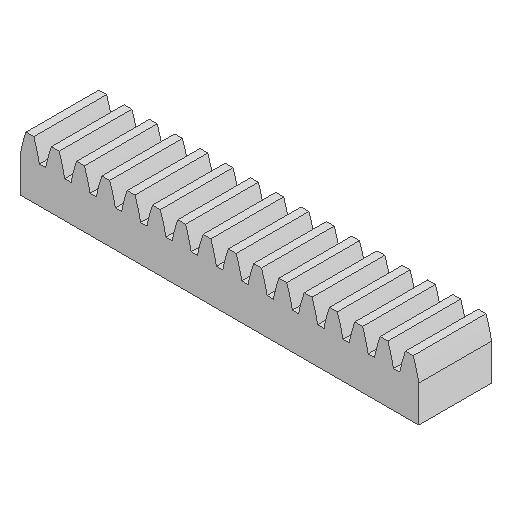
# Autodesk Inventor part: 1p10 DP3 gear attachment
Saved by Autodesk Inventor 2023 (Build 270158000, 158)
## iProperties
Created: 2023-03-02
Part Number: 1p10 DP3 gear attachment
Material: Generic
Document SubType Name: Modeling
Designer: Ethan Ko
Density: 1 g/cm^3
Appearance: Default
Author: Ethan Ko
Autodesk Inventor part; units mm, degrees
ref_plane "YZ Plane" through (0, 0, 0) normal (1, 0, 0) x (0, 1, 0)
ref_plane "XZ Plane" through (0, 0, 0) normal (0, 1, 0) x (-1, 0, 0)
ref_plane "XY Plane" through (0, 0, 0) normal (0, 0, 1) x (1, 0, 0)
sketch "Sketch1" plane through (0, 0, 0) normal (0, 0, 1) x (1, 0, 0)
  line L0 (0, 0) -> (1.071, 0)
  line L1 (0.5355, 0) -> (0.5355, -2.881)
  line L2 (0.5355, -2.881) -> (1.8385, -2.881)
  line L3 (1.8385, -2.881) -> (0.5355, -2.881)
  line L4 (0.5355, -2.881) -> (-0.7675, -2.881)
  arc A0 (0, 0) -> (-0.7675, -2.881) centre (20.5625, -7.0206) ccw
  arc A1 (1.8385, -2.881) -> (1.071, 0) centre (-19.4915, -7.0206) ccw
  line L5 (1.8385, -2.881) -> (2.7085, -2.881)
  line L6 (2.7085, -2.881) -> (5.3145, -2.881)
  line L7 (4.0115, -2.881) -> (4.0115, 0)
  line L8 (4.0115, 0) -> (3.476, 0)
  line L9 (4.0115, 0) -> (4.547, 0)
  arc A2 (3.476, 0) -> (2.7085, -2.881) centre (24.0385, -7.0206) ccw
  arc A3 (5.3145, -2.881) -> (4.547, 0) centre (-16.0155, -7.0206) ccw
  line L10 (5.3145, -2.881) -> (6.1845, -2.881)
  line L11 (6.1845, -2.881) -> (8.7905, -2.881)
  line L12 (7.4875, -2.881) -> (7.4875, 0)
  line L13 (7.4875, 0) -> (6.9515, 0)
  line L14 (7.4875, 0) -> (8.0235, 0)
  arc A4 (6.9515, 0) -> (6.1845, -2.881) centre (27.5152, -7.0172) ccw
  arc A5 (8.7905, -2.881) -> (8.0235, 0) centre (-12.5402, -7.0172) ccw
  line L15 (8.7905, -2.881) -> (9.6605, -2.881)
  line L16 (9.6605, -2.881) -> (12.2665, -2.881)
  line L17 (10.9635, -2.881) -> (10.9635, 0)
  line L18 (10.9635, 0) -> (10.4275, 0)
  line L19 (10.9635, 0) -> (11.4995, 0)
  arc A6 (10.4275, 0) -> (9.6605, -2.881) centre (30.9912, -7.0172) ccw
  arc A7 (12.2665, -2.881) -> (11.4995, 0) centre (-9.0642, -7.0172) ccw
  line L20 (-0.7675, -2.881) -> (-0.7675, -7.881)
  line L21 (12.2665, -2.881) -> (13.1365, -2.881)
  line L22 (13.1365, -2.881) -> (15.7425, -2.881)
  line L23 (14.4395, -2.881) -> (14.4395, 0)
  line L24 (14.4395, 0) -> (13.9035, 0)
  line L25 (14.4395, 0) -> (14.9755, 0)
  arc A8 (13.9035, 0) -> (13.1365, -2.881) centre (34.4672, -7.0172) ccw
  arc A9 (15.7425, -2.881) -> (14.9755, 0) centre (-5.5882, -7.0172) ccw
  line L26 (15.7425, -2.881) -> (16.6125, -2.881)
  line L27 (16.6125, -2.881) -> (19.2185, -2.881)
  line L28 (17.9155, -2.881) -> (17.9155, 0)
  line L29 (17.9155, 0) -> (17.3795, 0)
  line L30 (17.9155, 0) -> (18.4515, 0)
  arc A10 (17.3795, 0) -> (16.6125, -2.881) centre (37.9432, -7.0172) ccw
  arc A11 (19.2185, -2.881) -> (18.4515, 0) centre (-2.1122, -7.0172) ccw
  line L31 (19.2185, -2.881) -> (20.0885, -2.881)
  line L32 (20.0885, -2.881) -> (22.6945, -2.881)
  line L33 (21.3915, -2.881) -> (21.3915, 0)
  line L34 (21.3915, 0) -> (20.8555, 0)
  line L35 (21.3915, 0) -> (21.9275, 0)
  arc A12 (20.8555, 0) -> (20.0885, -2.881) centre (41.4192, -7.0172) ccw
  arc A13 (22.6945, -2.881) -> (21.9275, 0) centre (1.3638, -7.0172) ccw
  line L36 (22.6945, -2.881) -> (23.5645, -2.881)
  line L37 (23.5645, -2.881) -> (26.1705, -2.881)
  line L38 (24.8675, -2.881) -> (24.8675, 0)
  line L39 (24.8675, 0) -> (24.3315, 0)
  line L40 (24.8675, 0) -> (25.4035, 0)
  arc A14 (24.3315, 0) -> (23.5645, -2.881) centre (44.8952, -7.0172) ccw
  arc A15 (26.1705, -2.881) -> (25.4035, 0) centre (4.8398, -7.0172) ccw
  line L41 (26.1705, -2.881) -> (27.0405, -2.881)
  line L42 (27.0405, -2.881) -> (29.6465, -2.881)
  line L43 (29.6465, -2.881) -> (30.5165, -2.881)
  line L44 (30.5165, -2.881) -> (33.1225, -2.881)
  line L45 (33.1225, -2.881) -> (33.9925, -2.881)
  line L46 (33.9925, -2.881) -> (36.5985, -2.881)
  line L47 (36.5985, -2.881) -> (37.4685, -2.881)
  line L48 (37.4685, -2.881) -> (40.0745, -2.881)
  line L49 (40.0745, -2.881) -> (40.9445, -2.881)
  line L50 (40.9445, -2.881) -> (43.5505, -2.881)
  line L51 (43.5505, -2.881) -> (44.4205, -2.881)
  line L52 (44.4205, -2.881) -> (47.0265, -2.881)
  line L53 (47.0265, -2.881) -> (47.8965, -2.881)
  line L54 (47.8965, -2.881) -> (50.5025, -2.881)
  line L55 (50.5025, -2.881) -> (51.3725, -2.881)
  line L56 (51.3725, -2.881) -> (53.9785, -2.881)
  line L57 (53.9785, -2.881) -> (53.9785, -7.881)
  line L58 (53.9785, -7.881) -> (-0.7675, -7.881)
  line L59 (28.3435, -2.881) -> (28.3435, 0)
  line L60 (31.8195, -2.881) -> (31.8195, 0)
  line L61 (31.8195, 0) -> (31.2835, 0)
  line L62 (35.2955, -2.881) -> (35.2955, 0)
  line L63 (35.2955, 0) -> (34.7595, 0)
  line L64 (38.7715, -2.881) -> (38.7715, 0)
  line L65 (38.7715, 0) -> (38.2355, 0)
  line L66 (42.2475, -2.881) -> (42.2475, 0)
  line L67 (42.2475, 0) -> (41.7115, 0)
  line L68 (45.7235, -2.881) -> (45.7235, 0)
  line L69 (45.7235, 0) -> (45.1875, 0)
  line L70 (49.1995, -2.881) -> (49.1995, 0)
  line L71 (49.1995, 0) -> (48.6635, 0)
  line L72 (52.6755, -2.881) -> (52.6755, 0)
  line L73 (52.6755, 0) -> (52.1395, 0)
  line L74 (52.6755, 0) -> (53.2115, 0)
  line L75 (49.1995, 0) -> (49.7355, 0)
  line L76 (45.7235, 0) -> (46.2595, 0)
  line L77 (42.2475, 0) -> (42.7835, 0)
  line L78 (38.7715, 0) -> (39.3075, 0)
  line L79 (35.2955, 0) -> (35.8315, 0)
  line L80 (31.8195, 0) -> (32.3555, 0)
  line L81 (28.3435, 0) -> (28.8795, 0)
  line L82 (28.3435, 0) -> (27.8075, 0)
  arc A16 (27.8075, 0) -> (27.0405, -2.881) centre (48.3712, -7.0172) ccw
  arc A17 (29.6465, -2.881) -> (28.8795, 0) centre (8.3158, -7.0172) ccw
  arc A18 (31.2835, 0) -> (30.5165, -2.881) centre (51.8472, -7.0172) ccw
  arc A19 (33.1225, -2.881) -> (32.3555, 0) centre (11.7918, -7.0172) ccw
  arc A20 (34.7595, 0) -> (33.9925, -2.881) centre (55.3232, -7.0172) ccw
  arc A21 (36.5985, -2.881) -> (35.8315, 0) centre (15.2678, -7.0172) ccw
  arc A22 (38.2355, 0) -> (37.4685, -2.881) centre (58.7992, -7.0172) ccw
  arc A23 (40.0745, -2.881) -> (39.3075, 0) centre (18.7438, -7.0172) ccw
  arc A24 (41.7115, 0) -> (40.9445, -2.881) centre (62.2752, -7.0172) ccw
  arc A25 (43.5505, -2.881) -> (42.7835, 0) centre (22.2198, -7.0172) ccw
  arc A26 (45.1875, 0) -> (44.4205, -2.881) centre (65.7512, -7.0172) ccw
  arc A27 (47.0265, -2.881) -> (46.2595, 0) centre (25.6958, -7.0172) ccw
  arc A28 (48.6635, 0) -> (47.8965, -2.881) centre (69.2272, -7.0172) ccw
  arc A29 (50.5025, -2.881) -> (49.7355, 0) centre (29.1718, -7.0172) ccw
  arc A30 (52.1395, 0) -> (51.3725, -2.881) centre (72.7032, -7.0172) ccw
  arc A31 (53.9785, -2.881) -> (53.2115, 0) centre (32.6478, -7.0172) ccw
  dimension "d0" = 1.071
  dimension "d1" = 2.881
  dimension "d3" = 1.303
  dimension "d4" = 1.303
  dimension "d5" = 21.728
  dimension "d6" = 21.728
  dimension "d7" = 0.87
  dimension "d8" = 2.606
  dimension "d9" = 0.5355
  dimension "d10" = 0.5355
  dimension "d11" = 21.728
  dimension "d12" = 21.728
  dimension "d13" = 0.87
  dimension "d14" = 2.606
  dimension "d15" = 0.536
  dimension "d16" = 0.536
  dimension "d17" = 21.728
  dimension "d18" = 21.728
  dimension "d19" = 0.87
  dimension "d20" = 2.606
  dimension "d21" = 0.536
  dimension "d22" = 0.536
  dimension "d23" = 21.728
  dimension "d24" = 21.728
  dimension "d25" = 5
  dimension "d27" = 0.87
  dimension "d28" = 2.606
  dimension "d29" = 0.536
  dimension "d30" = 0.536
  dimension "d31" = 21.728
  dimension "d32" = 21.728
  dimension "d33" = 0.87
  dimension "d34" = 2.606
  dimension "d35" = 0.536
  dimension "d36" = 0.536
  dimension "d37" = 21.728
  dimension "d38" = 21.728
  dimension "d39" = 0.87
  dimension "d40" = 2.606
  dimension "d41" = 0.536
  dimension "d42" = 0.536
  dimension "d43" = 21.728
  dimension "d44" = 21.728
  dimension "d45" = 0.87
  dimension "d46" = 2.606
  dimension "d47" = 0.536
  dimension "d48" = 0.536
  dimension "d49" = 21.728
  dimension "d50" = 21.728
  dimension "d51" = 0.87
  dimension "d52" = 2.606
  dimension "d53" = 0.87
  dimension "d54" = 2.606
  dimension "d55" = 0.87
  dimension "d56" = 2.606
  dimension "d57" = 0.87
  dimension "d58" = 2.606
  dimension "d59" = 0.87
  dimension "d60" = 2.606
  dimension "d61" = 0.87
  dimension "d62" = 2.606
  dimension "d63" = 0.87
  dimension "d64" = 2.606
  dimension "d65" = 0.87
  constraints: 166 end point, 64 point on circle, 32 centre point, 32 horizontal, 21 point on line, 16 midpoint, 16 vertical, 12 perpendicular, 1 collinear
  measures "d0" distance of L0.start L0.end
  measures "d1" distance of L1.start L1.end
  measures "d3" distance of L1.end L2.end
  measures "d4" distance of L1.end L4.end
  measures "d5" radius of A0
  measures "d6" radius of A1
  measures "d7" distance of L2.end L5.end
  measures "d8" distance of L5.end L6.end
  measures "d9" distance of L7.end L8.end
  measures "d10" distance of L7.end L9.end
  measures "d11" radius of A2
  measures "d12" radius of A3
  measures "d13" distance of L6.end L10.end
  measures "d14" distance of L10.end L11.end
  measures "d15" distance of L12.end L13.end
  measures "d16" distance of L12.end L14.end
  measures "d17" radius of A4
  measures "d18" radius of A5
  measures "d19" distance of L11.end L15.end
  measures "d20" distance of L15.end L16.end
  measures "d21" distance of L17.end L18.end
  measures "d22" distance of L17.end L19.end
  measures "d23" radius of A6
  measures "d24" radius of A7
  measures "d25" distance of L4.end L20.end
  measures "d27" distance of L16.end L21.end
  measures "d28" distance of L21.end L22.end
  measures "d29" distance of L23.end L24.end
  measures "d30" distance of L23.end L25.end
  measures "d31" radius of A8
  measures "d32" radius of A9
  measures "d33" distance of L22.end L26.end
  measures "d34" distance of L26.end L27.end
  measures "d35" distance of L28.end L29.end
  measures "d36" distance of L28.end L30.end
  measures "d37" radius of A10
  measures "d38" radius of A11
  measures "d39" distance of L27.end L31.end
  measures "d40" distance of L31.end L32.end
  measures "d41" distance of L33.end L34.end
  measures "d42" distance of L33.end L35.end
  measures "d43" radius of A12
  measures "d44" radius of A13
  measures "d45" distance of L32.end L36.end
  measures "d46" distance of L36.end L37.end
  measures "d47" distance of L38.end L39.end
  measures "d48" distance of L38.end L40.end
  measures "d49" radius of A14
  measures "d50" radius of A15
  measures "d51" distance of L37.end L41.end
  measures "d52" distance of L41.end L42.end
  measures "d53" distance of L42.end L43.end
  measures "d54" distance of L43.end L44.end
  measures "d55" distance of L44.end L45.end
  measures "d56" distance of L45.end L46.end
  measures "d57" distance of L46.end L47.end
  measures "d58" distance of L47.end L48.end
  measures "d59" distance of L48.end L49.end
  measures "d60" distance of L49.end L50.end
  measures "d61" distance of L50.end L51.end
  measures "d62" distance of L51.end L52.end
  measures "d63" distance of L52.end L53.end
  measures "d64" distance of L53.end L54.end
  measures "d65" distance of L54.end L55.end
extrude "Extrusion1" add sketch "Sketch1" along normal blind 10
sketch "Sketch3" plane through (-0.7675, -7.881, 0) normal (0, -1, 0) x (1, 0, 0)
  circle A0 centre (27.373, 5) radius 3.5
  line L0 (54.746, 0) -> (54.746, 10) projected
  line L1 (0, 0) -> (54.746, 0) projected
  point P0 (0.7675, 0)
  dimension "d104" = 7
  dimension "d105" = 27.373
  dimension "d106" = 5
  constraints: 1 centre point
  measures "d104" diameter of A0
  measures "d105" distance from line of L0 A0.centre
  measures "d106" distance from line of L1 A0.centre
extrude "Extrusion3" cut sketch "Sketch3" against normal blind 3
body "Solid1"
